CJMCU-219 INA219 v13_v2 (Autodesk Fusion 360 design; units mm, degrees)
Autodesk Fusion 360 part; units mm, degrees
note: some values were not read from the file. Set by a fixed rule: which sketch regions a step uses.
sketch "Sketch1" plane through (0, 0, 0) normal (0, 1, 0) x (1, 0, 0)
  line L0 (0, 0) -> (25, 0)
  line L1 (25, 0) -> (25, 22.3)
  line L2 (25, 22.3) -> (0, 22.3)
  line L3 (0, 22.3) -> (0, 0)
  dimension "d1" = 25
  dimension "d2" = 22.3
  constraint horizontal L0
  constraint vertical L1
  constraint horizontal L2
  constraint vertical L3
  constraint coincident L0.start L3.end
  measures "d1" distance of L0.start L0.end
  measures "d2" distance of L0.start L2.end
extrude "Extrude1" add sketch "Sketch1" along normal blind 1.5
fillet "Fillet1" radius 2 4 edges at (25, 0.75, 0) (25, 0.75, -22.3) (0, 0.75, -22.3) (0, 0.75, 0)
sketch "Sketch2" plane through (0, 1.5, 0) normal (0, 1, 0) x (-1, 0, 0)
  arc A0 (0, -2) -> (-2, 0) centre (-2, -2) ccw
  line L0 (-2, 0) -> (-23, 0)
  arc A1 (-23, 0) -> (-25, -2) centre (-23, -2) ccw
  line L1 (-25, -2) -> (-25, -20.3)
  arc A2 (-25, -20.3) -> (-23, -22.3) centre (-23, -20.3) ccw
  line L2 (-23, -22.3) -> (-2, -22.3)
  arc A3 (-2, -22.3) -> (0, -20.3) centre (-2, -20.3) ccw
  line L3 (0, -20.3) -> (0, -2)
  line L4 (0, 0) -> (-2.25, 0)
  line L5 (-2.25, 0) -> (-2.2498, -2.55)
  circle A4 centre (-2.2498, -2.55) radius 1.25
  line L6 (-2.2498, -2.55) -> (-2.2499, -1.275)
  line L7 (-2.2498, -2.55) -> (-2.2498, -19.8)
  circle A5 centre (-2.2498, -19.8) radius 1.25
  line L8 (0, 0) -> (-6.5, 0)
  line L9 (-6.5, 0) -> (-6.5, -0.4982)
  circle A6 centre (-6.44, -2.9975) radius 0.45
  line L10 (-6.44, -2.9975) -> (-9.04, -2.9948)
  circle A7 centre (-9.04, -2.9948) radius 0.45
  line L11 (-9.04, -2.9948) -> (-11.64, -2.9944)
  circle A8 centre (-11.64, -2.9944) radius 0.45
  line L12 (0, 0) -> (-10.75, 0)
  line L13 (-10.75, 0) -> (-10.75, -19)
  circle A9 centre (-10.75, -19) radius 0.6
  line L14 (-9.2, -15.4) -> (-15.7, -15.4)
  line L15 (-15.7, -15.4) -> (-15.7, -12.1)
  line L16 (-15.7, -12.1) -> (-9.2, -12.1)
  line L17 (-9.2, -12.1) -> (-9.2, -15.4)
  line L18 (-3, -9.5) -> (-4.5, -9.5)
  line L19 (-4.5, -9.5) -> (-4.5, -7.5)
  line L20 (-4.5, -7.5) -> (-3, -7.5)
  line L21 (-3, -7.5) -> (-3, -9.5)
  line L22 (-5.5, -9.5) -> (-7, -9.5)
  line L23 (-7, -9.5) -> (-7, -7.5)
  line L24 (-7, -7.5) -> (-5.5, -7.5)
  line L25 (-5.5, -7.5) -> (-5.5, -9.5)
  line L26 (-8, -9.5) -> (-9.5, -9.5)
  line L27 (-9.5, -9.5) -> (-9.5, -7.5)
  line L28 (-9.5, -7.5) -> (-8, -7.5)
  line L29 (-8, -7.5) -> (-8, -9.5)
  line L30 (-14, -7.5) -> (-10.9513, -7.5)
  line L31 (-10.9513, -7.5) -> (-10.9513, -9.2569)
  line L32 (-10.9513, -9.2569) -> (-14, -9.2569)
  line L33 (-14, -9.2569) -> (-14, -7.5)
  line L34 (-17, -10) -> (-19, -10)
  line L35 (-19, -10) -> (-19, -8.5)
  line L36 (-19, -8.5) -> (-17, -8.5)
  line L37 (-17, -8.5) -> (-17, -10)
  line L38 (-17, -7.5) -> (-19, -7.5)
  line L39 (-19, -7.5) -> (-19, -6)
  line L40 (-19, -6) -> (-17, -6)
  line L41 (-17, -6) -> (-17, -7.5)
  line L42 (-11.64, -2.9944) -> (-14.24, -2.9944)
  line L43 (-14.24, -2.9944) -> (-16.84, -2.9944)
  line L44 (-16.84, -2.9944) -> (-19.44, -2.9944)
  circle A10 centre (-14.24, -2.9944) radius 0.45
  circle A11 centre (-16.84, -2.9944) radius 0.45
  circle A12 centre (-19.44, -2.9944) radius 0.45
  dimension "d6" = 2.25
  dimension "d7" = 2.55
  dimension "d8" = 2.5
  dimension "d9" = 17.25
  dimension "d10" = 2.5
  dimension "d11" = 6.5
  dimension "d12" = 2.5
  dimension "d13" = 0.9
  dimension "d14" = 6.5
  dimension "d15" = 2.6
  dimension "d16" = 0.9
  dimension "d17" = 2.6
  dimension "d18" = 0.9
  dimension "d22" = 10.75
  dimension "d23" = 19
  dimension "d24" = 1.2
  dimension "d28" = 2.6
  dimension "d29" = 2.6
  dimension "d30" = 2.6
  dimension "d31" = 0.9
  dimension "d32" = 0.9
  dimension "d33" = 0.9
  constraint coincident L4.start L8.start
  constraint coincident L5.end A4.centre
  constraint parallel L5 L6
  constraint vertical L7
  constraint coincident L7.end A5.centre
  constraint perpendicular L8 L9
  constraint coincident A6.centre L10.start
  constraint coincident L10.end A7.centre
  constraint coincident L11.end A8.centre
  constraint vertical L13
  constraint coincident L13.end A9.centre
  constraint horizontal L14
  constraint vertical L15
  constraint horizontal L16
  constraint vertical L17
  constraint horizontal L18
  constraint vertical L19
  constraint horizontal L20
  constraint vertical L21
  constraint horizontal L22
  constraint vertical L23
  constraint horizontal L24
  constraint vertical L25
  constraint horizontal L26
  constraint vertical L27
  constraint horizontal L28
  constraint vertical L29
  constraint horizontal L30
  constraint vertical L31
  constraint horizontal L32
  constraint vertical L33
  constraint horizontal L34
  constraint vertical L35
  constraint horizontal L36
  constraint vertical L37
  constraint horizontal L38
  constraint vertical L39
  constraint horizontal L40
  constraint vertical L41
  constraint horizontal L42
  constraint horizontal L43
  constraint horizontal L44
  constraint coincident L42.end L43.start
  constraint coincident L43.end L44.start
  constraint coincident L44.end A12.centre
  measures "d6" distance of L4.start L4.end
  measures "d7" distance of L4.end L5.end
  measures "d8" diameter of A4
  measures "d9" distance of L5.end L7.end
  measures "d10" diameter of A5
  measures "d11" distance of L4.start L8.end
  measures "d12" distance of L9.end A6.centre
  measures "d13" diameter of A6
  measures "d14" horizontal distance of L4.start L8.end
  measures "d15" distance of A6.centre L10.end
  measures "d16" diameter of A7
  measures "d17" distance of L10.end L11.end
  measures "d18" diameter of A8
  measures "d22" distance of L4.start L12.end
  measures "d23" distance of L12.end L13.end
  measures "d24" diameter of A9
  measures "d28" distance of L11.end L42.end
  measures "d29" distance of L42.end L43.end
  measures "d30" distance of L43.end L44.end
  measures "d31" diameter of A10
  measures "d32" diameter of A11
  measures "d33" diameter of A12
extrude "Extrude2" cut sketch "Sketch2" against normal blind 5 contours L5 A4 L6 L7 | L5 A4 L6 L7 | A5 | A9
ref_plane "WorkPlane1" through (12.5, 0.75, -11.15) normal (-1, 0, 0) x (0, 0, 1)
mirror "Mirror1" about plane through (12.5, 0.75, -11.15) normal (-1, 0, 0) of "Extrude2"
extrude "Extrude3" add sketch "Sketch2" along normal blind 1 contours L13 L14 L16 L17 | L13 L14 L15 L16 | L18 L19 L20 L21 | L22 L23 L24 L25 | L26 L27 L28 L29 | L30 L31 L32 L33 | L34 L35 L36 L37 | L38 L39 L40 L41
fillet "Fillet2" radius 0.6 12 edges at (9.2, 1.5, -13.75) (15.7, 1.5, -13.75) (8.75, 1.5, -7.5) (8.75, 1.5, -9.5) (6.25, 1.5, -7.5) (6.25, 1.5, -9.5) (3.75, 1.5, -9.5) (3.75, 1.5, -7.5) (19, 1.5, -9.25) (17, 1.5, -9.25) (17, 1.5, -6.75) (19, 1.5, -6.75)
extrude "Extrude4" cut sketch "Sketch2" against normal blind 4 contours A6 | L10 A7 L11 | L10 A7 L11 | L11 A8 L42 | L11 A8 L42 | L42 L43 A10 | L42 L43 A10 | L43 L44 A11 | L43 L44 A11 | A12
scale "Maßstab1" factor 0.9 about (3.4998, 1.5, -19.8) bodies 1
